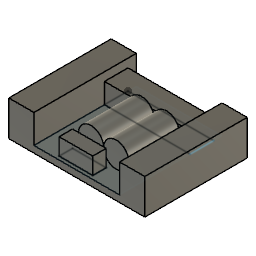
driver (Autodesk Fusion 360 design; units mm, degrees)
Autodesk Fusion 360 part; units mm, degrees
note: some values were not read from the file. Set by a fixed rule: which sketch regions a step uses.
sketch "Sketch1" plane through (0, 0, 0) normal (0, 0, 1) x (1, 0, 0)
  line L0 (40.5, -30.5) -> (-40.5, -30.5)
  line L1 (-40.5, -30.5) -> (-40.5, 30.5)
  line L2 (-40.5, 30.5) -> (40.5, 30.5)
  line L3 (40.5, 30.5) -> (40.5, -30.5)
  line L4 (40.5, -30.5) -> (-40.5, 30.5) construction
  line L5 (-40.5, -30.5) -> (40.5, 30.5) construction
  dimension "d1" = 81
  dimension "d2" = 61
  constraint horizontal L0
  constraint perpendicular L0 L1
  constraint parallel L0 L2
  constraint parallel L1 L3
  constraint coincident L4 origin
  constraint coincident L5 origin
  measures "d1" distance of L1.end L2.end
  measures "d2" distance of L0.end L1.end
extrude "Extrude1" add sketch "Sketch1" along normal blind 4 makes body 1
sketch "Sketch2" plane through (0, 0, 4) normal (0, 0, 1) x (-1, 0, 0)
  line L0 (-40.5, -30.5) -> (40.5, -30.5)
  line L1 (40.5, -30.5) -> (40.5, 30.5)
  line L2 (40.5, 30.5) -> (-40.5, 30.5)
  line L3 (-40.5, 30.5) -> (-40.5, -30.5)
  line L4 (40.5, -30.5) -> (25.5, -30.5)
  line L5 (25.5, -30.5) -> (25.5, 30.5)
  line L6 (25.5, 30.5) -> (40.5, 30.5)
  line L7 (40.5, 30.5) -> (40.5, -30.5)
  line L8 (0, -30.5) -> (0, 30) construction
  line L9 (-25.5, -30.5) -> (-25.5, 30.5)
  line L10 (-40.5, -30.5) -> (-25.5, -30.5)
  line L11 (-40.5, 30.5) -> (-40.5, -30.5)
  line L12 (-25.5, 30.5) -> (-40.5, 30.5)
  dimension "d5" = 15
  constraint horizontal L4
  constraint vertical L5
  constraint horizontal L6
  constraint vertical L7
  constraint coincident L0.end L1.start
  constraint midpoint L0 L8.start
  constraint perpendicular L0 L8
  constraint symmetric L0.end L8 L0.start
  constraint symmetric L4.end L8 L9.start
  constraint symmetric L5.end L8 L9.end
  constraint symmetric L1.end L8 L2.end
  measures "d5" distance of L0.end L4.end
extrude "Extrude2" add sketch "Sketch2" along normal blind 17 contours L0 L2 L3 L9 L10 L11 L12 | L0 L1 L2 L4 L5 L6 L7 bodies 1
sketch "Sketch3" plane through (0, 0, 4) normal (0, 0, 1) x (-1, 0, 0)
  line L0 (-25.5, 30.5) -> (-25.5, -30.5)
  line L1 (-25.5, -30.5) -> (25.5, -30.5)
  line L2 (25.5, -30.5) -> (25.5, 30.5)
  line L3 (25.5, 30.5) -> (-25.5, 30.5)
  line L4 (12.5, 28.5) -> (-7.5, 28.5)
  line L5 (-7.5, 28.5) -> (-7.5, 20.5)
  line L6 (-7.5, 20.5) -> (12.5, 20.5)
  line L7 (12.5, 20.5) -> (12.5, 28.5)
  line L8 (25.5, -25.5) -> (-25.5, -25.5)
  line L9 (-25.5, -25.5) -> (-25.5, -11.5)
  line L10 (-25.5, -11.5) -> (25.5, -11.5)
  line L11 (25.5, -11.5) -> (25.5, -25.5)
  dimension "d8" = 20
  dimension "d9" = 8
  dimension "d10" = 2
  dimension "d11" = 18
  dimension "d12" = 14
  dimension "d13" = 5
  constraint horizontal L4
  constraint vertical L5
  constraint horizontal L6
  constraint vertical L7
  constraint horizontal L8
  constraint vertical L9
  constraint horizontal L10
  constraint vertical L11
  constraint coincident L2 L8.start
  measures "d8" distance of L4.start L4.end
  measures "d9" distance of L4.start L6.end
  measures "d10" distance of L3 L4
  measures "d11" distance of L0 L5
  measures "d12" distance of L8.start L10.end
  measures "d13" distance of L1 L8
extrude "Extrude3" add sketch "Sketch3" along normal blind 10 contours L4 L5 L6 L7 bodies 1
extrude "Extrude4" add sketch "Sketch3" along normal blind 12 contours L0 L2 L8 L9 L10 L11 bodies 1
sketch "Sketch5" plane through (0, 11.5, 0) normal (0, -1, 0) x (1, 0, 0)
  line L0 (-25.5, 4) -> (25.5, 4)
  line L1 (25.5, 4) -> (25.5, 16)
  line L2 (25.5, 16) -> (-25.5, 16)
  line L3 (-25.5, 16) -> (-25.5, 4)
  circle A0 centre (11.5, 11.7785) radius 7.5
  circle A1 centre (-3.5, 11.7785) radius 7.5
  dimension "d18" = 15
  dimension "d19" = 14
  dimension "d20" = 15
  measures "d18" diameter of A0
  measures "d19" distance of L1 A0.centre
  measures "d20" diameter of A1
extrude "Extrude5" add sketch "Sketch5" along normal blind 30 separate body contours L2 A1 | L2 A1 | L2 A0 | L2 A0 makes body 2 at (-10.9631, -8.5, 12.5217)
